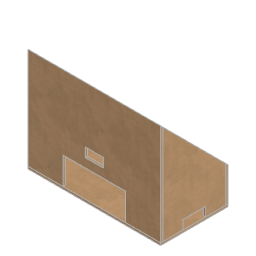
caret_llsif_controller_v3 (Autodesk Fusion 360 design; units mm, degrees)
Autodesk Fusion 360 part; units mm, degrees
sketch "Right Panel" plane through (0, 0, 0) normal (1, 0, 0) x (0, 1, 0)
  line L0 (0, 0) -> (352.026, 0)
  line L1 (0, 0) -> (0, 352.026)
  line L2 (352.026, 0) -> (0, 352.026)
  line L3 (0, 0) -> (0, -203.2)
  line L4 (0, -203.2) -> (112.513, -203.2)
  line L5 (352.026, 0) -> (352.026, -203.2)
  line L6 (352.026, -203.2) -> (239.513, -203.2)
  line L7 (239.513, -203.2) -> (239.513, -152.4)
  line L8 (112.513, -203.2) -> (112.513, -152.4)
  line L9 (239.513, -152.4) -> (112.513, -152.4)
  dimension "d16" = 352.026
  dimension "d17" = 352.026
  dimension "d18" = 203.2
  dimension "d19" = 112.513
  dimension "d20" = 203.2
  dimension "d21" = 112.513
  dimension "d22" = 50.8
  dimension "d24" = 50.8
  constraint coincident L0.start L1.start
  constraint horizontal L0
  constraint perpendicular L0 L1
  constraint perpendicular L0 L3
  constraint perpendicular L3 L4
  constraint perpendicular L0 L5
  constraint perpendicular L5 L6
  constraint perpendicular L6 L7
  constraint perpendicular L4 L8
  measures "d16" distance of L0.start L0.end
  measures "d17" distance of L0.start L1.end
  measures "d18" distance of L0.start L3.end
  measures "d19" distance of L3.end L4.end
  measures "d20" distance of L0.end L5.end
  measures "d21" distance of L5.end L6.end
  measures "d22" distance of L6.end L7.end
  measures "d24" distance of L4.end L8.end
sketch "Back Panel" plane through (0, 0, 0) normal (0, 1, 0) x (1, 0, 0)
  line L0 (0, 0) -> (717.55, 0)
  line L1 (0, -352.026) -> (0, 0)
  line L2 (0, 0) -> (717.55, 0)
  line L3 (717.55, 0) -> (717.55, 203.2)
  line L4 (717.55, 203.2) -> (0, 203.2)
  line L5 (0, 203.2) -> (0, 0)
  line L6 (0, 0) -> (717.55, 0)
  line L7 (717.55, 0) -> (717.55, -352.026)
  line L8 (717.55, -352.026) -> (0, -352.026)
  line L9 (0, -352.026) -> (0, 0)
  line L10 (358.775, 203.2) -> (358.775, 0)
  line L11 (358.775, 203.2) -> (184.15, 203.2)
  line L12 (358.775, 203.2) -> (533.4, 203.2)
  line L13 (184.15, 203.2) -> (539.75, 203.2)
  line L14 (358.775, 203.2) -> (184.15, 203.2)
  line L15 (184.15, 203.2) -> (184.15, 50.8)
  line L16 (184.15, 50.8) -> (358.775, 50.8)
  line L17 (358.775, 50.8) -> (358.775, 203.2)
  line L18 (358.775, 203.2) -> (533.4, 203.2)
  line L19 (533.4, 203.2) -> (533.4, 50.8)
  line L20 (533.4, 50.8) -> (358.775, 50.8)
  line L21 (358.775, 50.8) -> (358.775, 203.2)
  line L22 (358.775, 0) -> (307.975, 0)
  line L23 (307.975, 0) -> (307.975, -50.8)
  line L24 (307.975, -50.8) -> (358.775, -50.8)
  line L25 (358.775, -50.8) -> (358.775, 0)
  line L26 (358.775, -50.8) -> (409.575, -50.8)
  line L27 (409.575, -50.8) -> (409.575, 0)
  line L28 (409.575, 0) -> (358.775, 0)
  line L29 (358.775, 0) -> (358.775, -50.8)
  dimension "d25" = 717.55
  dimension "d26" = 352.026
  dimension "d27" = 203.2
  dimension "d29" = 717.55
  dimension "d30" = 352.026
  dimension "d44" = 174.625
  dimension "d45" = 152.4
  dimension "d46" = 174.625
  dimension "d47" = 152.4
  dimension "d48" = 50.8
  dimension "d49" = 50.8
  dimension "d50" = 50.8
  constraint horizontal L0
  constraint vertical L1
  constraint coincident L0.start L1.end
  constraint horizontal L2
  constraint vertical L3
  constraint horizontal L4
  constraint vertical L5
  constraint horizontal L6
  constraint vertical L7
  constraint horizontal L8
  constraint vertical L9
  constraint midpoint L4 L10.start
  constraint midpoint L0 L10.end
  constraint perpendicular L10 L11
  constraint perpendicular L10 L12
  constraint horizontal L13
  constraint horizontal L14
  constraint vertical L15
  constraint horizontal L16
  constraint vertical L17
  constraint horizontal L18
  constraint vertical L19
  constraint horizontal L20
  constraint vertical L21
  constraint horizontal L22
  constraint vertical L23
  constraint horizontal L24
  constraint vertical L25
  constraint horizontal L26
  constraint vertical L27
  constraint horizontal L28
  constraint vertical L29
  measures "d25" distance of L0.start L0.end
  measures "d26" distance of L0.start L1.start
  measures "d27" distance of L0.start L4.end
  measures "d29" distance of L0.start L0.end
  measures "d30" distance of L0.start L1.start
  measures "d44" distance of L10.start L11.end
  measures "d45" distance of L10.start L16.end
  measures "d46" distance of L10.start L12.end
  measures "d47" distance of L10.start L16.end
  measures "d48" distance of L10.end L22.end
  measures "d49" distance of L24.end L26.end
  measures "d50" distance of L24.end L10.end
sketch "Left Panel" plane through (0, 0, 0) normal (1, 0, 0) x (0, 1, 0)
  line L0 (352.026, 0, 717.55) -> (0, 352.026, 717.55)
  line L1 (352.026, -203.2, 717.55) -> (239.513, -203.2, 717.55)
  line L2 (0, -203.2, 717.55) -> (112.513, -203.2, 717.55)
  line L3 (352.026, 0, 717.55) -> (352.026, -203.2, 717.55)
  line L4 (0, 0, 717.55) -> (0, -203.2, 717.55)
  line L5 (239.513, -152.4, 717.55) -> (112.513, -152.4, 717.55)
  line L6 (0, 0, 717.55) -> (0, 352.026, 717.55)
  line L7 (0, 0, 717.55) -> (352.026, 0, 717.55)
  line L8 (239.513, -203.2, 717.55) -> (239.513, -152.4, 717.55)
  line L9 (112.513, -203.2, 717.55) -> (112.513, -152.4, 717.55)
  dimension "d31" = 352.026
  dimension "d32" = 352.026
  dimension "d33" = 203.2
  dimension "d34" = 112.513
  dimension "d35" = 203.2
  dimension "d36" = 112.513
  dimension "d37" = 50.8
  dimension "d38" = 50.8
sketch "Front Panel" plane through (0, 0, 0) normal (0, 1, 0) x (1, 0, 0)
  line L0 (184.15, 203.2, 352.026) -> (539.75, 203.2, 352.026)
  line L1 (358.775, 50.8, 352.026) -> (358.775, 203.2, 352.026)
  line L2 (409.575, 0, 352.026) -> (358.775, 0, 352.026)
  line L3 (0, 0, 352.026) -> (717.55, 0, 352.026)
  line L4 (358.775, 0, 352.026) -> (307.975, 0, 352.026)
  line L5 (358.775, 203.2, 352.026) -> (184.15, 203.2, 352.026)
  line L6 (0, 0, 352.026) -> (717.55, 0, 352.026)
  line L7 (358.775, 203.2, 352.026) -> (184.15, 203.2, 352.026)
  line L8 (717.55, 0, 352.026) -> (717.55, 203.2, 352.026)
  line L9 (358.775, 203.2, 352.026) -> (533.4, 203.2, 352.026)
  line L10 (358.775, 50.8, 352.026) -> (358.775, 203.2, 352.026)
  line L11 (358.775, 203.2, 352.026) -> (533.4, 203.2, 352.026)
  line L12 (0, 203.2, 352.026) -> (0, 0, 352.026)
  line L13 (717.55, 203.2, 352.026) -> (0, 203.2, 352.026)
  line L14 (358.775, 203.2, 352.026) -> (358.775, 0, 352.026)
  line L15 (0, 0, 352.026) -> (717.55, 0, 352.026)
  line L16 (358.775, 203.2, 352.026) -> (438.15, 203.2, 352.026)
  line L17 (438.15, 203.2, 352.026) -> (438.15, 50.8, 352.026)
  line L18 (438.15, 50.8, 352.026) -> (358.775, 50.8, 352.026)
  line L19 (358.775, 50.8, 352.026) -> (358.775, 203.2, 352.026)
  line L20 (358.775, 203.2, 352.026) -> (184.15, 203.2, 352.026)
  line L21 (184.15, 203.2, 352.026) -> (184.15, 50.8, 352.026)
  line L22 (184.15, 50.8, 352.026) -> (358.775, 50.8, 352.026)
  line L23 (358.775, 50.8, 352.026) -> (358.775, 203.2, 352.026)
  dimension "d53" = 717.55
  dimension "d54" = 203.2
  dimension "d55" = 717.55
  dimension "d57" = 152.4
  dimension "d60" = 50.8
  dimension "d61" = 79.375
  dimension "d62" = 152.4
  dimension "d63" = 174.625
  dimension "d64" = 152.4
sketch "Bottom_Ghost" plane through (0, 0, 0) normal (0, 0, 1) x (1, 0, 0)
  line L0 (0, 0) -> (717.55, 0)
  line L1 (717.55, 0) -> (717.55, 352.026)
  line L2 (717.55, 352.026) -> (0, 352.026)
  line L3 (0, 352.026) -> (0, 0)
  dimension "d65" = 717.55
  dimension "d66" = 352.026
  constraint horizontal L0
  constraint vertical L1
  constraint horizontal L2
  constraint vertical L3
  constraint coincident L0.start L3.end
  measures "d65" distance of L0.start L0.end
  measures "d66" distance of L0.start L2.end
sketch "Bottom" plane through (0, 0, 0) normal (0, 0, 1) x (1, 0, 0)
  line L0 (717.55, 352.026, -203.2) -> (0, 352.026, -203.2)
  line L1 (0, 0, -203.2) -> (717.55, 0, -203.2)
  line L2 (717.55, 0, -203.2) -> (717.55, 352.026, -203.2)
  line L3 (0, 352.026, -203.2) -> (0, 0, -203.2)
  dimension "d67" = 717.55
  dimension "d68" = 352.026
extrude "Extrude1" add sketch "Back Panel" against normal blind 12.7 contours L0 L2 L4 L5 L6 L10 L15 L16 L22 | L0 L1 L2 L6 L7 L8 L9 L23 L24 L26 L27 | L0 L2 L3 L4 L6 L10 L13 L19 L20 L28 makes body 1
extrude "Extrude2" add sketch "Left Panel" along normal blind 12.7 separate body contours L0 L6 L7 | L1 L2 L3 L4 L5 L7 L8 L9 in plane through (717.55, 0, 0) normal (1, 0, 0) makes body 2
extrude "Extrude3" add sketch "Front Panel" along normal blind 12.7 separate body contours L3 L4 L6 L12 L13 L14 L15 L21 L22 | L0 L2 L3 L6 L8 L9 L11 L13 L14 L15 L17 L18 in plane through (0, 352.026, 0) normal (0, 1, 0) makes body 3
extrude "Extrude4" add sketch "Right Panel" against normal blind 12.7 separate body makes body 4
extrude "Extrude5" add sketch "Bottom" against normal blind 12.7 separate body contours L0 L1 L2 L3 in plane through (0, 0, -203.2) normal (0, 0, 1) makes body 5
extrude "Extrude6" add 1 faces at (239.1833, -8.4667, 352.026) along direction (0, 0, 1) blind 12.7 on bodies 1 bodies 1
chamfer "Chamfer1" distance 12.7 angle 45 1 edges at (358.775, 0, 364.726) on bodies 1
extrude "Extrude7" add 1 faces at (717.55, -8.4667, 171.1849) along direction (1, 0, 0) blind 12.7 on bodies 1 bodies 1
extrude "Extrude8" add 1 faces at (0, -8.4667, 171.1849) along direction (-1, 0, 0) blind 12.7 on bodies 1 bodies 1
extrude "Extrude9" add 1 faces at (717.55, 356.2593, -67.7333) along direction (1, 0, 0) blind 12.7 on bodies 3 bodies 3
extrude "Extrude10" add 1 faces at (0, 356.2593, -135.4667) along direction (-1, 0, 0) blind 12.7 on bodies 3 bodies 3
extrude "Extrude11" add 1 faces at (239.1833, 352.026, -211.6667) along direction (0, 1, 0) blind 12.7 on bodies 5 bodies 5
extrude "Extrude12" add 1 faces at (0, 243.1507, -207.4333) along direction (-1, 0, 0) blind 12.7 on bodies 5 bodies 5
extrude "Extrude13" add 1 faces at (230.7167, 0, -211.6667) along direction (0, -1, 0) blind 12.7 on bodies 5 bodies 5
extrude "Extrude14" add 1 faces at (717.55, 238.9174, -207.4333) along direction (1, 0, 0) blind 12.7 on bodies 5 bodies 5
chamfer "Chamfer2" distance 12.7 angle 45 1 edges at (358.775, 364.726, 0) on bodies 3
equation "button_board_height = 19.6 in"
equation "h_pc_box = 8 in"
equation "tri_sides = button_board_height * sin(45 deg)"
equation "d16 = tri_sides"
equation "d17 = tri_sides"
equation "d18 = h_pc_box"
equation "d19 = ( tri_sides / 2 ) - 2.5 in"
equation "d20 = h_pc_box"
equation "d21 = ( tri_sides / 2 ) - 2.5 in"
equation "d25 = button_board_width"
equation "d26 = tri_sides"
equation "d27 = h_pc_box"
equation "button_board_width = 28.25 in"
equation "d29 = button_board_width"
equation "d30 = tri_sides"
equation "d31 = tri_sides"
equation "d32 = tri_sides"
equation "d33 = h_pc_box"
equation "d34 = ( tri_sides / 2 ) - 2.5 in"
equation "d35 = h_pc_box"
equation "d36 = ( tri_sides / 2 ) - 2.5 in"
equation "w_pc_back_access = 13.75 in"
equation "h_pc_back_access = 6 in"
equation "d44 = w_pc_back_access / 2"
equation "d45 = h_pc_back_access"
equation "d46 = w_pc_back_access / 2"
equation "d47 = h_pc_back_access"
equation "d53 = button_board_width"
equation "d54 = h_pc_box"
equation "d55 = button_board_width"
equation "d57 = h_pc_back_access"
equation "d61 = 10 in - 6.875 in"
equation "d65 = button_board_width"
equation "d66 = tri_sides"
equation "d67 = button_board_width"
equation "d68 = tri_sides"
equation "d69 = -wood_thickness"
equation "d71 = wood_thickness"
equation "d73 = wood_thickness"
equation "d75 = -wood_thickness"
equation "d77 = -wood_thickness"
equation "d79 = wood_thickness"
equation "d81 = wood_thickness"
equation "d82 = wood_thickness"
equation "wood_thickness = 0.5 in"
equation "d85 = wood_thickness"
equation "d87 = wood_thickness"
equation "d89 = wood_thickness"
equation "d91 = wood_thickness"
equation "d93 = wood_thickness"
equation "d95 = wood_thickness"
equation "d97 = wood_thickness"
equation "d99 = wood_thickness"
named bodies: "Back"
